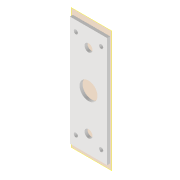
# Autodesk Inventor part: 40_microfluidic_chip_lightsheet_layer2_v0
Saved by Autodesk Inventor 2022 (Build 260153000, 153)
## iProperties
Created: 2021-12-21
Part Number: 40_microfluidic_chip_lightsheet_layer2_v0
Material: Generisch
Document SubType Name: Modeling
Designer: diederichbenedict
Density: 1 g/cm^3
Appearance: Vorgabe
Author: diederichbenedict
Autodesk Inventor part; units mm, degrees
ref_plane "YZ Plane" through (0, 0, 0) normal (1, 0, 0) x (0, 1, 0)
ref_plane "XZ Plane" through (0, 0, 0) normal (0, 1, 0) x (-1, 0, 0)
ref_plane "XY Plane" through (0, 0, 0) normal (0, 0, 1) x (1, 0, 0)
ref_plane "Arbeitsebene1" through (0, 0, 0) normal (0, 0, 1) x (1, 0, 0)
sketch "Skizze1" plane through (0, 0, 0) normal (0, 0, 1) x (1, 0, 0)
  circle A0 centre (0, -25) radius 2.5 projected
  circle A1 centre (0, 25) radius 2.5 projected
  line L0 (12.5, -37) -> (12.5, 37) projected
  line L1 (12.5, 37) -> (-12.5, 37) projected
  line L2 (-12.5, 37) -> (-12.5, -37) projected
  line L3 (-12.5, -37) -> (12.5, -37) projected
  circle A2 centre (8.5, -30) radius 1.4 projected
  circle A3 centre (-8.5, -30) radius 1.4 projected
  circle A4 centre (-8.5, 30) radius 1.4 projected
  circle A5 centre (8.5, 30) radius 1.4 projected
  circle A6 centre (0, 0) radius 6
  circle A7 centre (0, 25) radius 2.7
  circle A8 centre (0, -25) radius 2.7
  line L4 (-9.25, 9.25) -> (9.25, 9.25) projected
  line L5 (9.25, 9.25) -> (9.25, -9.25) projected
  line L6 (9.25, -9.25) -> (-9.25, -9.25) projected
  line L7 (-9.25, -9.25) -> (-9.25, 9.25) projected
  point P0 (0.75, -9.25)
  point P1 (-0.75, -9.25)
  point P2 (-0.75, 9.25)
  point P3 (0.75, 9.25)
  point P4 (0.75, 5.9529)
  point P5 (-0.75, 5.9529)
  point P6 (0.75, -5.9529)
  point P7 (-0.75, -5.9529)
  dimension "d0" = 12
  dimension "d4" = 0.2
  dimension "d5" = 0.2
  constraints: 4 point on circle, 3 centre point, 1 coincident
  measures "d0" diameter of A6
  measures "d4" radial gap between concentric circles of A0 A8
  measures "d5" radial gap between concentric circles of A7 A1
extrude "Extrusion1" add sketch "Skizze1" along normal blind 2 contours L3 L2 L1 L0 | L4 L5 L6 L7
sketch "Skizze2" plane through (0, 0, 0) normal (0, 0, -1) x (-1, 0, 0)
  line L0 (-9, -9) -> (-9, 9) projected
  line L1 (9, -9) -> (-9, -9) projected
  line L2 (9, 9) -> (9, -9) projected
  line L3 (-9, 9) -> (9, 9) projected
  line L4 (9.5, -9.5) -> (-9.5, -9.5)
  line L5 (-9.5, -9.5) -> (-9.5, 9.5)
  line L6 (-9.5, 9.5) -> (9.5, 9.5)
  line L7 (9.5, 9.5) -> (9.5, -9.5)
  point P0 (0, 0)
  dimension "d6" = 0.5
  constraints: 8 end point, 3 other
  measures "d6" distance between parallel lines of L2 L7
